# Autodesk Inventor part: Welle
Saved by Autodesk Inventor 2016 (Build 200138000, 138)
## iProperties
Created: 2016-03-29
Part Number: Welle
Material: Steel
Document SubType Name: Modeling
Designer: 4ndreas
Density: 7.85 g/cm^3
Appearance: Steel
Mass: 3.13407 g
Surface Area: 4.19245 cm^2
Volume: 0.399244 cm^3
CustomPartVersion: 1
Author: 4ndreas
Autodesk Inventor part; units mm, degrees
ref_plane "Startebene" through (0, 0, 0) normal (1, 0, 0) x (0, 1, 0)
ref_plane "XZ Plane" through (0, 0, 0) normal (0, 1, 0) x (-1, 0, 0)
ref_plane "XY Plane" through (0, 0, 0) normal (0, 0, 1) x (1, 0, 0)
sketch "Hauptskizze" plane through (0, 0, 0) normal (0, 0, 1) x (1, 0, 0)
  line L0 (0, 0) -> (32, 0)
  line L1 (0, 0) -> (0, 2)
  line L2 (0, 2) -> (16, 2)
  line L3 (32, 2) -> (32, 0)
  line L4 (16, 2) -> (32, 2)
  dimension "d3" = 4
  dimension "d5" = 4
  constraints: 10 end point, 2 horizontal, 2 vertical
  measures "d3" diameter of L2 L0
  measures "d5" diameter of L4 L0
revolve "Umdrehung1" add sketch "Hauptskizze" angle 360 about axis through (0, 0, 0) along (1, 0, 0)
chamfer "Fase3" distance 0.5 angle 45 1 edges at (0, -2, 0) measured on face at (10.6667, 1.9741, -0.3208)
chamfer "Fase2" distance 0.5 angle 45 1 edges at (32, -2, 0) measured on face at (26.6667, 1.9935, -0.1609)
